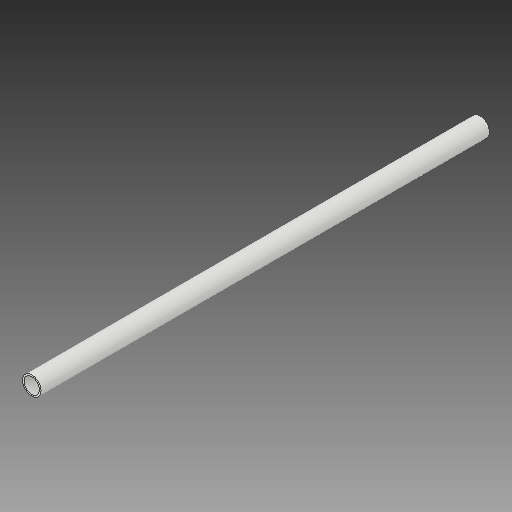
# Autodesk Inventor part: Main Rod
Saved by Autodesk Inventor 2018 (Build 220112000, 112)
## iProperties
Created: 2018-04-18
Part Number: Main Rod
Material: PVC-Piping
Document SubType Name: Modeling
Designer: 232963
Density: 1.4 g/cm^3
Appearance: Smooth - White
Mass: 76.6868 g
Surface Area: 618.313 cm^2
Volume: 54.7763 cm^3
Author: 232963
Autodesk Inventor part; units mm, degrees
ref_plane "YZ Plane" through (0, 0, 0) normal (1, 0, 0) x (0, 1, 0)
ref_plane "XZ Plane" through (0, 0, 0) normal (0, 1, 0) x (-1, 0, 0)
ref_plane "XY Plane" through (0, 0, 0) normal (0, 0, 1) x (1, 0, 0)
sketch "Sketch1" plane through (0, 0, 0) normal (0, 0, 1) x (1, 0, 0)
  circle A0 centre (0, 0) radius 8.763
  circle A1 centre (0, 0) radius 10.541
  dimension "d0" = 17.526
  dimension "d1" = 1.778
  constraints: 2 centre point, 2 coincident
  measures "d0" diameter of A0
  measures "d1" radial gap between concentric circles of A0 A1
extrude "Extrusion1" add sketch "Sketch1" along normal blind 508
body "Solid1"
